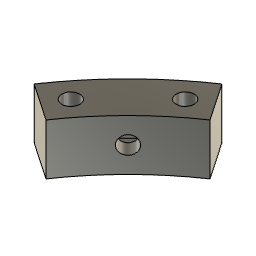
sphere2_block v5 (Autodesk Fusion 360 design; units mm, degrees)
Autodesk Fusion 360 part; units mm, degrees
sketch "Skizze1" plane through (0, 0, 0) normal (0, 0, 1) x (1, 0, 0)
  circle A0 centre (0, 0) radius 65 construction
  line L0 (-66.7503, 52.1511) -> (89.6233, -70.0214) construction
  line L1 (-51.5684, 66.0045) -> (50.4838, -64.6164) construction
  line L2 (-86.5753, 0) -> (92.1282, 0) construction
  line L3 (0, 84.3443) -> (0, -71.5181) construction
  circle A1 centre (0, 0) radius 60.6
  circle A2 centre (0, 0) radius 69.4
  line L4 (-42.8236, 63.013) -> (41.6736, -61.3209)
  line L5 (-61.3482, 41.6922) -> (84.2724, -57.2715)
  circle A3 centre (-51.2207, 40.018) radius 1.75
  circle A4 centre (-40.018, 51.2207) radius 1.75
  line L6 (-91.6282, 91.6282) -> (70.0913, -70.0913) construction
  line L7 (-102.9597, -11.0359) -> (6.8047, 98.7286) construction
  point P0 (-51.2207, 40.018)
  point P1 (-40.018, 51.2207)
  point P2 (-51.2207, 40.018)
  point P3 (-40.018, 51.2207)
  point P4 (-45.9619, 45.9619)
  dimension "d1" = 130
  dimension "d2" = 38
  dimension "d3" = 38
  dimension "d4" = 121.2
  dimension "d5" = 138.8
  dimension "d6" = 34.2
  dimension "d7" = 34.2
  dimension "d10" = 3.5
  dimension "d11" = 3.5
  dimension "d12" = 45
  constraint coincident A0.centre A1.centre
  constraint coincident A0.centre L0
  constraint coincident A0.centre L1
  constraint horizontal L2
  constraint coincident A0.centre L2
  constraint vertical L3
  constraint coincident A0.centre L3
  constraint coincident A0.centre L4
  constraint coincident A0.centre L5
  constraint coincident A0 P2
  constraint coincident L0 P2
  constraint coincident A0 P3
  constraint coincident L1 P3
  constraint coincident P2 P0
  constraint coincident P3 P1
  constraint coincident A0.centre L6
  constraint coincident L6 P4
  constraint coincident A0 P4
  constraint perpendicular L6 L7
  constraint coincident P4 L7
  measures "d1" diameter of A0
  measures "d2" angle of L1 L3
  measures "d3" angle of L0 L2
  measures "d4" diameter of A1
  measures "d5" diameter of A2
  measures "d6" angle of L3 L4
  measures "d7" angle of L2 L5
  measures "d10" diameter of A4
  measures "d11" diameter of A3
  measures "d12" angle of L2 L6
ref_plane "Arbeitsebene1" through (0, 0, 0) normal (0.707107, 0.707107, 0) x (-0.707107, 0.707107, 0)
sketch "Skizze3" plane through (0, 0, 0) normal (0.707107, 0.707107, 0) x (-0.707107, 0.707107, 0)
  line L0 (65, 53.8628) -> (65, -35) construction
  point P0 (65, 0)
  constraint vertical L0
  constraint coincident L0 P0
ref_plane "Arbeitsebene2" through (-45.9619, 45.9619, 0) normal (0.707107, -0.707107, 0) x (0.707107, 0.707107, 0)
sketch "Skizze4" plane through (-45.9619, 45.9619, 0) normal (0.707107, -0.707107, 0) x (0.707107, 0.707107, 0)
  line L0 (0, 44.1227) -> (0, -35) construction
  line L1 (53.181, 0) -> (-38.9604, 0) construction
  line L2 (51.233, 5) -> (-51.6226, 5) construction
  line L3 (1.7032, 2.05) -> (3.4064, 5)
  line L4 (3.4064, 5) -> (1.7032, 7.95)
  line L5 (1.7032, 7.95) -> (-1.7032, 7.95)
  line L6 (-1.7032, 7.95) -> (-3.4064, 5)
  line L7 (-3.4064, 5) -> (-1.7032, 2.05)
  line L8 (-1.7032, 2.05) -> (1.7032, 2.05)
  line L9 (3.4064, 7.95) -> (-3.4064, 7.95)
  line L10 (-3.4064, 7.95) -> (-3.4064, 5)
  line L11 (-3.4064, 5) -> (3.4064, 5)
  line L12 (3.4064, 5) -> (3.4064, 7.95)
  circle A0 centre (0, 5) radius 1.75
  point P0 (0, 5)
  dimension "d13" = 5
  dimension "d15" = 5.9
  dimension "d28" = 3.5
  constraint vertical L0
  constraint coincident L0 origin
  constraint horizontal L1
  constraint coincident origin L1
  constraint horizontal L2
  constraint coincident L2 P0
  constraint coincident L0 P0
  constraint horizontal L9
  constraint vertical L10
  constraint horizontal L11
  constraint vertical L12
  constraint coincident L6.end L7.start
  constraint coincident L3.end L4.start
  constraint coincident L5 L9.start
  constraint coincident P0 A0.centre
  measures "d13" distance of L1 L2
  measures "d15" distance of L5 L8
  measures "d28" diameter of A0
extrude "Extrusion1" add sketch "Skizze1" along normal blind 10 contours A1 A2 L4 L5 picked at (-47.8032, 46.0094)
extrude "Extrusion2" cut sketch "Skizze4" along normal mid plane 2.8
ref_plane "Arbeitsebene3" through (0, 0, 5) normal (0, 0, 1) x (1, 0, 0)
sketch "Skizze5" plane through (0, 0, 5) normal (0, 0, 1) x (1, 0, 0)
  line L0 (-43.0431, 55.0926) -> (33.9956, -43.5124) construction
  line L1 (-63.2817, 49.4411) -> (43.7853, -34.2088) construction
  line L2 (-70, 0) -> (67.6704, 0) construction
  line L3 (0, 69.2816) -> (0, -27.82) construction
  circle A0 centre (0, 0) radius 65 construction
  line L4 (-36.8485, 49.9727) -> (-37.3524, 53.3415)
  line L5 (-37.3524, 53.3415) -> (-40.5219, 54.5896)
  line L6 (-40.5219, 54.5896) -> (-43.1875, 52.4687)
  line L7 (-43.1875, 52.4687) -> (-42.6836, 49.0999)
  line L8 (-42.6836, 49.0999) -> (-39.5141, 47.8518)
  line L9 (-39.5141, 47.8518) -> (-36.8485, 49.9727)
  line L10 (-47.8518, 39.5141) -> (-49.0999, 42.6836)
  line L11 (-49.0999, 42.6836) -> (-52.4687, 43.1875)
  line L12 (-52.4687, 43.1875) -> (-54.5896, 40.5219)
  line L13 (-54.5896, 40.5219) -> (-53.3415, 37.3524)
  line L14 (-53.3415, 37.3524) -> (-49.9727, 36.8485)
  line L15 (-49.9727, 36.8485) -> (-47.8518, 39.5141)
  point P0 (-40.018, 51.2207)
  point P1 (-51.2207, 40.018)
  point P2 (-40.018, 51.2207)
  point P3 (-51.2207, 40.018)
  dimension "d21" = 38
  dimension "d22" = 38
  dimension "d23" = 130
  dimension "d24" = 5.9
  dimension "d25" = 5.9
  constraint coincident A0.centre L0
  constraint coincident A0.centre L1
  constraint horizontal L2
  constraint coincident A0.centre L2
  constraint vertical L3
  constraint coincident A0.centre L3
  constraint coincident A0.centre origin
  constraint coincident L0 P2
  constraint coincident A0 P2
  constraint coincident L1 P3
  constraint coincident A0 P3
  constraint coincident P2 P0
  constraint coincident P3 P1
  measures "d21" angle of L0 L3
  measures "d22" angle of L1 L2
  measures "d23" diameter of A0
  measures "d24" distance of L12 L15
  measures "d25" distance of L6 L9
extrude "Extrusion3" cut sketch "Skizze5" along normal mid plane 2.8
extrude "Extrusion4" cut sketch "Skizze4" along normal mid plane 30 contours L11 A0 | L11 A0
